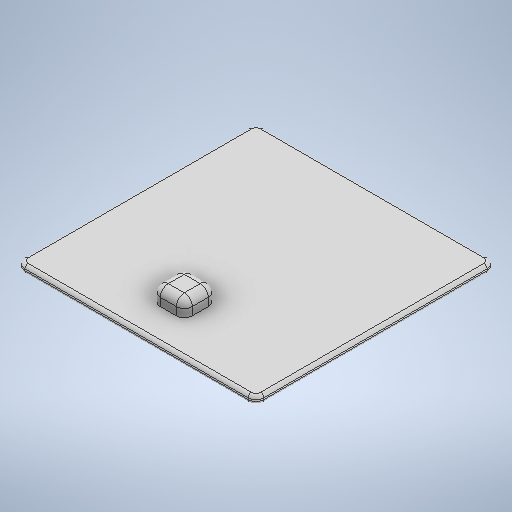
# Autodesk Inventor part: slider
Saved by Autodesk Inventor 2026.1 (Build 301233000, 233)
## iProperties
Created: 2026-05-31
Part Number: slider
Material: Generic
Document SubType Name: Modeling
Designer: chris
Density: 1 g/cm^3
Appearance: Default
Author: chris
Autodesk Inventor part; units mm, degrees
ref_plane "YZ Plane" through (0, 0, 0) normal (1, 0, 0) x (0, 1, 0)
ref_plane "XZ Plane" through (0, 0, 0) normal (0, 1, 0) x (-1, 0, 0)
ref_plane "XY Plane" through (0, 0, 0) normal (0, 0, 1) x (1, 0, 0)
sketch "Sketch1" plane through (0, 0, 0) normal (0, 1, 0) x (-1, 0, 0)
  line L0 (75, 75) -> (-75, 75)
  line L1 (-75, 75) -> (-75, -75)
  line L2 (-75, -75) -> (75, -75)
  line L3 (75, -75) -> (75, 75)
  line L4 (75, 75) -> (-75, -75) construction
  line L5 (-75, 75) -> (75, -75) construction
  point P0 (0, 0)
  dimension "d0" = 150
  dimension "d1" = 150
  constraints: 12 end point, 2 midpoint, 2 parallel, 1 horizontal, 1 perpendicular
  measures "d0" distance of L2.end L1.end
  measures "d1" distance of L1.end L0.end
extrude "Extrusion1" add sketch "Sketch1" along normal blind 5
sketch "Sketch2" plane through (0, 5, 0) normal (0, 1, 0) x (1, 0, 0)
  line L0 (10, -55) -> (-10, -55)
  line L1 (-10, -55) -> (-10, -35)
  line L2 (-10, -35) -> (10, -35)
  line L3 (10, -35) -> (10, -55)
  line L4 (10, -55) -> (-10, -35) construction
  line L5 (-10, -55) -> (10, -35) construction
  line L6 (-75, -75) -> (75, -75) projected
  point P0 (0, 0)
  point P1 (0, -45)
  dimension "d4" = 20
  dimension "d5" = 20
  dimension "d6" = 20
  constraints: 12 end point, 2 midpoint, 2 parallel, 1 horizontal, 1 perpendicular
  measures "d4" distance of L1.end L2.end
  measures "d5" distance of L0.end L1.end
  measures "d6" distance between parallel lines of L0 L6
extrude "Extrusion2" add sketch "Sketch2" along normal blind 10
fillet "Fillet1" radius 5 12 edges at (75, 2.5, 75) (75, 2.5, -75) (-75, 2.5, 75) (-75, 2.5, -75) (10, 10, 55) (10, 10, 35) (-10, 10, 35) (-10, 10, 55) (-10, 15, 45) (0, 15, 55) (10, 15, 45) (0, 15, 35)
fillet "Fillet2" radius 2 16 edges at (73.5355, 5, -73.5355) (0, 5, -75) (-73.5355, 5, -73.5355) (-75, 5, 0) (-73.5355, 5, 73.5355) (0, 5, 75) (73.5355, 5, 73.5355) (75, 5, 0) (73.5355, 0, -73.5355) (0, 0, -75) (-73.5355, 0, -73.5355) (-75, 0, 0) (-73.5355, 0, 73.5355) (0, 0, 75) (73.5355, 0, 73.5355) (75, 0, 0)
body "Solid1"
